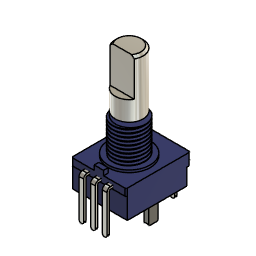
CUI_ACZ11BR2E-20FD1 (Autodesk Fusion 360 design; units mm, degrees)
Autodesk Fusion 360 part; units mm, degrees
sketch "Sketch1" plane through (0, 0, 0) normal (0, 0, 1) x (1, 0, 0) in component "Body"
  line L0 (5.85, -6.5) -> (-5.85, -6.5)
  line L1 (-5.85, -6.5) -> (-5.85, 7.25)
  line L2 (-5.85, 7.25) -> (5.85, 7.25)
  line L3 (5.85, 7.25) -> (5.85, -6.5)
  line L4 (5.85, -6.5) -> (-5.85, 7.25) construction
  line L5 (-5.85, -6.5) -> (5.85, 7.25) construction
  line L6 (0, 0.375) -> (0, 0) construction
  point P0 (0, 0.375)
  dimension "d1" = 11.7
  dimension "d2" = 7.25
  dimension "d3" = 6.5
  constraint horizontal L0
  constraint perpendicular L0 L1
  constraint parallel L0 L2
  constraint parallel L1 L3
  constraint coincident L4 P0
  constraint coincident L5 P0
  constraint coincident P0 L6.start
  constraint coincident L6.end origin
  constraint vertical L6
  measures "d1" distance of L1.end L2.end
  measures "d2" vertical distance of L6.end L2.end
  measures "d3" vertical distance of L6.end L0.start
extrude "Extrude1" add sketch "Sketch1" along normal blind 6 makes body 1 in component "Body"
sketch "Sketch2" plane through (0, 0, 6) normal (0, 0, 1) x (-1, 0, 0) in component "Body"
  line L0 (-5.85, -7.25) -> (5.85, -7.25)
  line L1 (5.85, -7.25) -> (5.85, 6.5)
  line L2 (5.85, 6.5) -> (-5.85, 6.5)
  line L3 (-5.85, 6.5) -> (-5.85, -7.25)
  circle A0 centre (0, 0) radius 4.5
  dimension "d6" = 9
  constraint coincident A0.centre origin
  measures "d6" diameter of A0
extrude "Extrude2" add sketch "Sketch2" along normal blind 0.5 contours A0 bodies 1 in component "Body"
sketch "Sketch3" plane through (0, 0, 6.5) normal (0, 0, 1) x (-1, 0, 0) in component "Body"
  circle A0 centre (0, 0) radius 4.5
  circle A1 centre (0, 0) radius 3.5
  dimension "d9" = 7
  constraint concentric A0 A1
  measures "d9" diameter of A1
extrude "Extrude3" add sketch "Sketch3" along normal blind 7 contours A1 bodies 1 in component "Body"
thread "Thread1" "ISO Metric profile 7.0 M7x0.75 6g" major diameter 6.908 minor diameter 6.0475 pitch 0.75 angle 60 modelled right hand crest width 0.1053 on face at (-3.4826, 0.3485, 11.1667) crest through (-3.454, 0, 6.3125) on bodies 1 in component "Body"
sketch "Sketch4" plane through (0, 0, 6) normal (0, 0, 1) x (-1, 0, 0) in component "Body"
  circle A0 centre (0, 0) radius 4.5
  line L0 (-5.85, -7.25) -> (5.85, -7.25)
  line L1 (5.85, -7.25) -> (5.85, 6.5)
  line L2 (5.85, 6.5) -> (-5.85, 6.5)
  line L3 (-5.85, 6.5) -> (-5.85, -7.25)
  line L4 (0, 0) -> (0, 6.5) construction
  line L5 (-1, 6.5) -> (1, 6.5)
  line L6 (1, 6.5) -> (1, 5.5)
  line L7 (1, 5.5) -> (-1, 5.5)
  line L8 (-1, 5.5) -> (-1, 6.5)
  line L9 (-1, 6.5) -> (1, 5.5) construction
  line L10 (1, 6.5) -> (-1, 5.5) construction
  point P0 (0, 6)
  dimension "d12" = 2
  dimension "d13" = 1
  dimension "d14" = 6
  constraint coincident A0.centre L4.start
  constraint midpoint L2 L4.end
  constraint horizontal L5
  constraint perpendicular L5 L6
  constraint parallel L5 L7
  constraint parallel L6 L8
  constraint coincident L9 P0
  constraint coincident L10 P0
  constraint coincident L4 P0
  measures "d12" distance of L6.end L7.end
  measures "d13" distance of L5.end L6.end
  measures "d14" distance of A0.centre P0
extrude "Extrude4" add sketch "Sketch4" along normal blind 1 contours L2 L5 L6 L7 L8 bodies 1 in component "Body"
sketch "Sketch6" plane through (-5.85, 0, 0) normal (-1, 0, 0) x (0, -1, 0) in component "Body"
  line L0 (-7.25, 0) -> (6.5, 0)
  line L1 (6.5, 0) -> (6.5, 6)
  line L2 (6.5, 6) -> (-7.25, 6)
  line L3 (-7.25, 6) -> (-7.25, 0)
  line L4 (-7.25, 4.5) -> (-7, 4.5)
  line L5 (-7, 4.5) -> (-7, 3.5)
  line L6 (-7, 3.5) -> (-6.5, 3.5)
  line L7 (-6.5, 3.5) -> (-6.5, 0)
  line L8 (-6.5, 0) -> (-7.25, 0)
  line L9 (-7.25, 0) -> (-7.25, 4.5)
  line L10 (6.5, 4.5) -> (6.25, 4.5)
  line L11 (6.25, 4.5) -> (6.25, 0)
  line L12 (6.25, 0) -> (6.5, 0)
  line L13 (6.5, 0) -> (6.5, 4.5)
  dimension "d18" = 1.5
  dimension "d19" = 1
  dimension "d20" = 0.25
  dimension "d21" = 0.75
  dimension "d22" = 0.25
  dimension "d23" = 4.5
  dimension "d24" = 4.5
  constraint coincident L3 L4.start
  constraint perpendicular L3 L4
  constraint perpendicular L4 L5
  constraint perpendicular L5 L6
  constraint coincident L0 L7.end
  constraint perpendicular L0 L7
  constraint perpendicular L3 L8
  constraint perpendicular L4 L9
  constraint coincident L1 L10.start
  constraint perpendicular L1 L10
  constraint coincident L0 L11.end
  constraint perpendicular L0 L11
  constraint coincident L0.end L1.start
  measures "d18" distance of L2.end L4.start
  measures "d19" distance of L4.end L5.end
  measures "d20" distance of L4.start L4.end
  measures "d21" horizontal distance of L4.start L6.end
  measures "d22" distance of L10.start L10.end
  measures "d23" distance of L4.start L0.start
  measures "d24" distance of L10.end L11.end
extrude "Extrude5" cut sketch "Sketch6" against normal through all contours L0 L3 L4 L5 L6 L7 L8 L9 | L0 L1 L10 L11 L12 L13 bodies 1 in component "Body"
fillet "Fillet1" radius 0.25 4 edges at (5.85, -6.5, 5.25) (-5.85, -6.5, 5.25) (5.85, 7.25, 5.25) (-5.85, 7.25, 5.25) on bodies 1 in component "Body"
sketch "Sketch1 (2)" plane through (0, 0, 13.5) normal (0, 0, 1) x (-1, 0, 0) in component "Shaft"
  spline S0 degree 3 poles (1.2545, 2.7513) (0.9045, 2.9407) (0.5206, 3.059) (-0.2814, 3.1449) (-0.692, 3.1077) (-1.4866, 2.8769) (-1.8618, 2.6817) (-2.5256, 2.1535) (-2.8055, 1.8225) (-3.1606, 1.1866) (-3.2707, 0.9073) (-3.4159, 0.3225) (-3.4491, 0.0192) (-3.4423, -0.2844) knots 0 0 0 0 0.119376 0.119376 0.241821 0.241821 0.367335 0.367335 0.495916 0.495916 0.585378 0.585378 0.676274 0.676274 0.676274 0.676274
  arc A0 (-3.4423, -0.2844) -> (-1.9674, -2.8389) centre (0, 0) ccw
  spline S1 degree 3 poles (-1.9674, -2.8389) (-1.5881, -3.0695) (-1.1679, -3.2246) (-0.3016, -3.3616) (0.1356, -3.346) (0.9687, -3.1486) (1.3575, -2.9725) (2.0363, -2.4858) (2.322, -2.183) (2.6866, -1.6004) (2.8011, -1.349) (2.9588, -0.8271) (3.0024, -0.5593) (3.0099, -0.2892) knots 0 0 0 0 0.133171 0.133171 0.263268 0.263268 0.39029 0.39029 0.514237 0.514237 0.596919 0.596919 0.678165 0.678165 0.678165 0.678165
  arc A1 (3.0099, -0.2892) -> (1.2545, 2.7513) centre (0, 0) ccw
  circle A2 centre (0, 0) radius 1.5
  dimension "d28" = 3
  constraint coincident A0.centre A1.centre
  measures "d28" diameter of A2
extrude "Extrude1'" add sketch "Sketch1 (2)" along normal blind 0.8 separate body contours A2 makes body 2 in component "Shaft"
sketch "Sketch2 (2)" plane through (0, 0, 14.3) normal (0, 0, 1) x (-1, 0, 0) in component "Shaft"
  circle A0 centre (0, 0) radius 1.5
  circle A1 centre (0, 0) radius 3
  dimension "d31" = 6
  constraint concentric A0 A1
  measures "d31" diameter of A1
extrude "Extrude2'" add sketch "Sketch2 (2)" along normal blind 12.2 contours A0 | A1 bodies 2 in component "Shaft"
chamfer "Chamfer1" distance 0.5 angle 45 1 edges at (2.797, 1.0848, 26.5) on bodies 2 in component "Shaft"
sketch "Sketch3 (2)" plane through (0, 0, 26.5) normal (0, 0, 1) x (-1, 0, 0) in component "Shaft"
  circle A0 centre (0, 0) radius 2.5
  circle A1 centre (0, 0) radius 3
  line L0 (2.5981, 1.5) -> (-2.5981, 1.5)
  line L1 (0, -3) -> (0, 1.5) construction
  arc A2 (2.5981, 1.5) -> (-2.5981, 1.5) centre (0, 0) ccw
  dimension "d35" = 4.5
  constraint coincident A1 L1.start
  constraint coincident L0 L1.end
  constraint perpendicular L0 L1
  constraint coincident A0.centre L1
  constraint coincident A1 L0.end
  constraint coincident A1 L0.start
  constraint horizontal L0
  constraint coincident A0.centre A1.centre
  measures "d35" distance of L1.start L1.end
extrude "Extrude3'" cut sketch "Sketch3 (2)" against normal blind 8 contours A0 L0 | A0 A1 L0 A2 picked at (0.2131, 1.8706) bodies 2 in component "Shaft"
sketch "Sketch1 (3)" plane through (0, -6.25, 0) normal (0, -1, 0) x (1, 0, 0) in component "Pins"
  line L0 (5.85, 0) -> (5.85, 4.5)
  line L1 (5.85, 4.5) -> (-5.85, 4.5)
  line L2 (-5.85, 4.5) -> (-5.85, 0)
  line L3 (-5.85, 0) -> (5.85, 0)
  line L4 (0.5, 4.75) -> (-0.5, 4.75)
  line L5 (-0.5, 4.75) -> (-0.5, 5.25)
  line L6 (-0.5, 5.25) -> (0.5, 5.25)
  line L7 (0.5, 5.25) -> (0.5, 4.75)
  line L8 (0.5, 4.75) -> (-0.5, 5.25) construction
  line L9 (-0.5, 4.75) -> (0.5, 5.25) construction
  line L10 (0, 6) -> (0, 0) construction
  point P0 (0, 5)
  dimension "d38" = 1
  dimension "d39" = 0.5
  dimension "d41" = 0.5
  constraint horizontal L4
  constraint perpendicular L4 L5
  constraint parallel L4 L6
  constraint parallel L5 L7
  constraint coincident L8 P0
  constraint coincident L9 P0
  constraint coincident L10.end origin
  constraint perpendicular L3 L10
  constraint coincident P0 L10
  measures "d38" distance of L5.end L6.end
  measures "d39" distance of L4.end L5.end
  measures "d41" distance of L1 P0
sketch "Sketch2 (3)" plane through (0, 0, 0) normal (1, 0, 0) x (0, 1, 0) in component "Pins"
  line L0 (0, 0) -> (-7.5, 0) construction
  line L1 (-7.5, -4) -> (-7.5, -3.9301)
  line L2 (-7.5, -3.9301) -> (-7.5, 4.5)
  arc A0 (-7, 5) -> (-7.5, 4.5) centre (-7, 4.5) ccw
  line L3 (-7, 4.5) -> (-7, 5) construction
  line L4 (-7, 4.5) -> (-7.5, 4.5) construction
  line L5 (-7, 5) -> (-6.25, 5)
  line L6 (-7, 5) -> (-7, 0) construction
  point P0 (-6.25, 5)
  point P1 (-6.25, 0)
  dimension "d42" = 7.5
  dimension "d43" = 4
  dimension "d44" = 90
  dimension "d45" = 0.5
  constraint coincident L0.start origin
  constraint horizontal L0
  constraint perpendicular L0 L1
  constraint perpendicular L0 L2
  constraint coincident P0 L5.end
  constraint horizontal L5
  constraint coincident L0 L6.end
  constraint perpendicular L0 L6
  constraint coincident A0.centre L6
  constraint coincident L0.end L2
  measures "d42" distance of L0.start L0.end
  measures "d43" distance of L0.end L1.start
  measures "d44" angle of L3 L4
  measures "d45" radius of A0
sweep "Sweep1" add profiles "Sketch1 (3)" path "Sketch2 (3)" along L1 L2 A0 L5 section 1 contours L4 L5 L6 L7 separate body makes body 3 in component "Pins"
fillet "Fillet1'" radius 0.5 2 edges at (0.5, -7.5, -4) (-0.5, -7.5, -4) on bodies 3 in component "Pins"
pattern_linear "R-Pattern1" count 3 spacing 2.5 along (1, 0, 0) both ways of bodies 3 makes body 4 at (-2.3333, -7.25, -0.8334) makes body 5 at (2.6667, -7.75, 1.8333) in component "Pins"
sketch "Sketch3 (3)" plane through (0, 6.5, 0) normal (0, 1, 0) x (-1, 0, 0) in component "Pins"
  line L0 (-5.85, 3.5) -> (-5.85, 0)
  line L1 (-5.85, 0) -> (5.85, 0)
  line L2 (5.85, 0) -> (5.85, 3.5)
  line L3 (5.85, 3.5) -> (-5.85, 3.5)
  line L4 (0, 0) -> (0, 3.5) construction
  line L5 (-2.5, 0) -> (-2.5, 3.5) construction
  line L6 (-2, 0.5) -> (-3, 0.5)
  line L7 (-3, 0.5) -> (-3, 1)
  line L8 (-3, 1) -> (-2, 1)
  line L9 (-2, 1) -> (-2, 0.5)
  line L10 (-2, 0.5) -> (-3, 1) construction
  line L11 (-3, 0.5) -> (-2, 1) construction
  point P0 (-2.5, 0.75)
  dimension "d58" = 2.5
  dimension "d59" = 1
  dimension "d60" = 0.5
  dimension "d61" = 0.75
  constraint coincident L4.start origin
  constraint midpoint L3 L4.end
  constraint coincident L1 L5.start
  constraint coincident L3 L5.end
  constraint perpendicular L3 L5
  constraint horizontal L6
  constraint perpendicular L6 L7
  constraint parallel L6 L8
  constraint parallel L7 L9
  constraint coincident L10 P0
  constraint coincident L11 P0
  constraint coincident L5 P0
  measures "d58" distance of L4.end L5.end
  measures "d59" distance of L7.end L8.end
  measures "d60" distance of L6.end L7.end
  measures "d61" distance of L5.start P0
sketch "Sketch4 (2)" plane through (0, 0, 0) normal (1, 0, 0) x (0, 1, 0) in component "Pins"
  line L0 (0, 0) -> (7, 0) construction
  line L1 (7, 0.25) -> (7, -4)
  arc A0 (7, 0.25) -> (6.5, 0.75) centre (6.5, 0.25) ccw
  line L2 (6.5, 0.25) -> (7, 0.25) construction
  line L3 (6.5, 0.25) -> (6.5, 0.75) construction
  point P0 (6.5, 0.75)
  point P1 (6.5, 0)
  dimension "d62" = 7
  dimension "d63" = 4
  dimension "d64" = 90
  dimension "d65" = 0.5
  constraint coincident L0.end L1
  constraint vertical L3
  constraint coincident L0.start origin
  constraint coincident L1.start A0.start
  constraint vertical L1
  constraint coincident P1 L0
  constraint coincident P0 A0.end
  measures "d62" distance of L0.start L0.end
  measures "d63" distance of L0.end L1.end
  measures "d64" angle of L2 L3
  measures "d65" radius of A0
sweep "Sweep2" add profiles "Sketch3 (3)" path "Sketch4 (2)" along A0 L1 section 1 contours L6 L7 L8 L9 separate body makes body 6 in component "Pins"
fillet "Fillet2" radius 0.5 2 edges at (3, 7, -4) (2, 7, -4) on bodies 6 in component "Pins"
pattern_linear "R-Pattern2" count 2 spacing 5 along (-1, 0, 0) of bodies 6 makes body 7 in component "Pins"
sketch "Sketch5" plane through (0, 0, 0) normal (0, 0, -1) x (1, 0, 0) in component "Pins"
  line L0 (-5.85, -6.5) -> (5.85, -6.5)
  line L1 (5.85, -6.5) -> (5.85, 6.25)
  line L2 (5.85, 6.25) -> (-5.85, 6.25)
  line L3 (-5.85, 6.25) -> (-5.85, -6.5)
  line L4 (5.85, 0) -> (-5.85, 0) construction
  line L5 (5.2, 1) -> (4.2, 1)
  line L6 (4.2, 1) -> (4.2, -1)
  line L7 (4.2, -1) -> (5.2, -1)
  line L8 (5.2, -1) -> (5.2, 1)
  line L9 (5.2, 1) -> (4.2, -1) construction
  line L10 (4.2, 1) -> (5.2, -1) construction
  line L11 (-5.2, 1) -> (-4.2, 1)
  line L12 (-4.2, 1) -> (-4.2, -1)
  line L13 (-4.2, -1) -> (-5.2, -1)
  line L14 (-5.2, -1) -> (-5.2, 1)
  line L15 (-5.2, 1) -> (-4.2, -1) construction
  line L16 (-4.2, 1) -> (-5.2, -1) construction
  line L17 (0, 0) -> (0, -6.5) construction
  point P0 (4.7, 0)
  point P1 (-4.7, 0)
  dimension "d78" = 1
  dimension "d79" = 2
  dimension "d80" = 9.4
  constraint coincident L1 L4.start
  constraint coincident L3 L4.end
  constraint perpendicular L3 L4
  constraint coincident L17.start L4
  constraint horizontal L5
  constraint perpendicular L5 L6
  constraint parallel L5 L7
  constraint parallel L6 L8
  constraint coincident L9 P0
  constraint coincident L10 P0
  constraint coincident L4 P0
  constraint horizontal L11
  constraint perpendicular L11 L12
  constraint parallel L11 L13
  constraint parallel L12 L14
  constraint coincident L15 P1
  constraint coincident L16 P1
  constraint coincident L4 P1
  constraint equal L7 L13
  constraint equal L6 L14
  constraint coincident L17.start origin
  constraint midpoint L0 L17.end
  constraint symmetric P0 P1 L17
  measures "d78" distance of L6.end L7.end
  measures "d79" distance of L5.end L6.end
  measures "d80" distance of P0 P1
extrude "Extrude1''" add sketch "Sketch5" along normal blind 4 separate body contours L5 L6 L7 L8 | L11 L12 L13 L14 makes body 8 at (5.2, 0.3333, -1.3333) makes body 9 at (-4.2, -0.3333, -1.3333) in component "Pins"
fillet "Fillet3" radius 0.25 4 edges at (4.7, -1, -4) (4.7, 1, -4) (-4.7, -1, -4) (-4.7, 1, -4) on bodies 8 9 in component "Pins"
component "Body" placed x (1, 0, 0) y (0, 1, 0) z (0, 0, 1) at (0, 0, 0)
component "Shaft" placed x (1, 0, 0) y (0, 1, 0) z (0, 0, 1) at (0, 0, 0)
component "Pins" placed x (1, 0, 0) y (0, 1, 0) z (0, 0, 1) at (0, 0, 0)
equation "d22 = d20"
